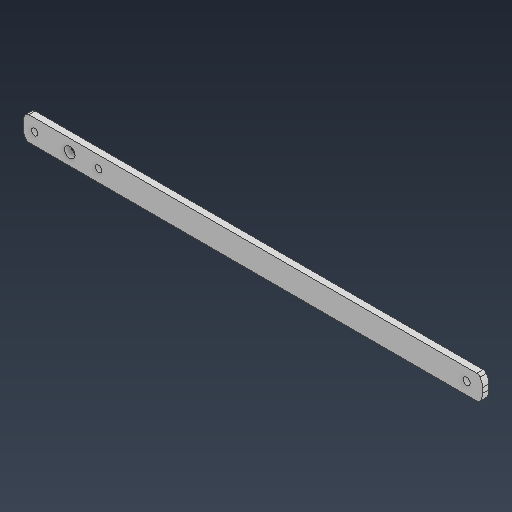
# Autodesk Inventor part: ДЛЯ ПОДВЕСА
Saved by Autodesk Inventor 2025 (Build 290162000, 162)
## iProperties
Created: 2025-03-11
Part Number: ДЛЯ ПОДВЕСА
Material: Типовые
Document SubType Name: Modeling
Designer: GameHD
Density: 1 g/cm^3
Appearance: По умолчанию
Author: GameHD
Autodesk Inventor part; units mm, degrees
ref_plane "YZ Plane" through (0, 0, 0) normal (1, 0, 0) x (0, 1, 0)
ref_plane "XZ Plane" through (0, 0, 0) normal (0, 1, 0) x (-1, 0, 0)
ref_plane "XY Plane" through (0, 0, 0) normal (0, 0, 1) x (1, 0, 0)
sketch "Эскиз1" plane through (0, 0, 0) normal (0, 0, 1) x (1, 0, 0)
  arc A0 (130.1731, 0.7623) -> (123.4106, 7.5248) centre (123.4106, 0.7623) ccw
  line L0 (-123.2839, 7.5248) -> (123.4106, 7.5248)
  arc A1 (-123.2839, 7.5248) -> (-130.0464, 0.7623) centre (-123.2839, 0.7623) ccw
  line L1 (-130.0464, -1.7127) -> (-130.0464, 0.7623)
  arc A2 (-130.0464, -1.7127) -> (-123.2839, -8.4752) centre (-123.2839, -1.7127) ccw
  line L2 (123.4106, -8.4752) -> (-123.2839, -8.4752)
  arc A3 (123.4106, -8.4752) -> (130.1731, -1.7127) centre (123.4106, -1.7127) ccw
  line L3 (130.1731, 0.7623) -> (130.1731, -1.7127)
  circle A4 centre (122.1731, -0.4752) radius 1.85
  circle A5 centre (-124.1763, -0.4762) radius 1.65
  circle A6 centre (-106.5766, -0.4757) radius 2.65
  circle A7 centre (-92.1769, -0.4756) radius 1.65
  line L4 (-73.2645, 4.044) -> (-78.5234, -4.9714)
  arc A8 (-71.5369, 4.044) -> (-73.2645, 4.044) centre (-72.4007, 3.5401) ccw
  line L5 (-66.2779, -4.9714) -> (-71.5369, 4.044)
  arc A9 (-67.1417, -6.4752) -> (-66.2779, -4.9714) centre (-67.1417, -5.4752) ccw
  line L6 (-77.6596, -6.4752) -> (-67.1417, -6.4752)
  arc A10 (-78.5234, -4.9714) -> (-77.6596, -6.4752) centre (-77.6596, -5.4752) ccw
  line L7 (-57.8267, 5.5248) -> (-68.3446, 5.5248)
  arc A11 (-56.9629, 4.0209) -> (-57.8267, 5.5248) centre (-57.8267, 4.5248) ccw
  line L8 (-62.2219, -4.9945) -> (-56.9629, 4.0209)
  arc A12 (-63.9495, -4.9945) -> (-62.2219, -4.9945) centre (-63.0857, -4.4906) ccw
  line L9 (-69.2084, 4.0209) -> (-63.9495, -4.9945)
  arc A13 (-68.3446, 5.5248) -> (-69.2084, 4.0209) centre (-68.3446, 4.5248) ccw
  line L10 (-54.634, 4.044) -> (-59.893, -4.9714)
  arc A14 (-52.9065, 4.044) -> (-54.634, 4.044) centre (-53.7703, 3.5401) ccw
  line L11 (-47.6475, -4.9714) -> (-52.9065, 4.044)
  arc A15 (-48.5113, -6.4752) -> (-47.6475, -4.9714) centre (-48.5113, -5.4752) ccw
  line L12 (-59.0292, -6.4752) -> (-48.5113, -6.4752)
  arc A16 (-59.893, -4.9714) -> (-59.0292, -6.4752) centre (-59.0292, -5.4752) ccw
  line L13 (-39.1963, 5.5248) -> (-49.7142, 5.5248)
  arc A17 (-38.3325, 4.0209) -> (-39.1963, 5.5248) centre (-39.1963, 4.5248) ccw
  line L14 (-43.5915, -4.9945) -> (-38.3325, 4.0209)
  arc A18 (-45.319, -4.9945) -> (-43.5915, -4.9945) centre (-44.4553, -4.4906) ccw
  line L15 (-50.578, 4.0209) -> (-45.319, -4.9945)
  arc A19 (-49.7142, 5.5248) -> (-50.578, 4.0209) centre (-49.7142, 4.5248) ccw
  line L16 (-36.0036, 4.044) -> (-41.2626, -4.9714)
  arc A20 (-34.2761, 4.044) -> (-36.0036, 4.044) centre (-35.1399, 3.5401) ccw
  line L17 (-29.0171, -4.9714) -> (-34.2761, 4.044)
  arc A21 (-29.8809, -6.4752) -> (-29.0171, -4.9714) centre (-29.8809, -5.4752) ccw
  line L18 (-40.3988, -6.4752) -> (-29.8809, -6.4752)
  arc A22 (-41.2626, -4.9714) -> (-40.3988, -6.4752) centre (-40.3988, -5.4752) ccw
  line L19 (-20.5659, 5.5248) -> (-31.0838, 5.5248)
  arc A23 (-19.7021, 4.0209) -> (-20.5659, 5.5248) centre (-20.5659, 4.5248) ccw
  line L20 (-24.9611, -4.9945) -> (-19.7021, 4.0209)
  arc A24 (-26.6886, -4.9945) -> (-24.9611, -4.9945) centre (-25.8249, -4.4906) ccw
  line L21 (-31.9476, 4.0209) -> (-26.6886, -4.9945)
  arc A25 (-31.0838, 5.5248) -> (-31.9476, 4.0209) centre (-31.0838, 4.5248) ccw
  line L22 (-17.3732, 4.044) -> (-22.6322, -4.9714)
  arc A26 (-15.6457, 4.044) -> (-17.3732, 4.044) centre (-16.5095, 3.5401) ccw
  line L23 (-10.3867, -4.9714) -> (-15.6457, 4.044)
  arc A27 (-11.2505, -6.4752) -> (-10.3867, -4.9714) centre (-11.2505, -5.4752) ccw
  line L24 (-21.7684, -6.4752) -> (-11.2505, -6.4752)
  arc A28 (-22.6322, -4.9714) -> (-21.7684, -6.4752) centre (-21.7684, -5.4752) ccw
  line L25 (-1.9355, 5.5248) -> (-12.4534, 5.5248)
  arc A29 (-1.0717, 4.0209) -> (-1.9355, 5.5248) centre (-1.9355, 4.5248) ccw
  line L26 (-6.3307, -4.9945) -> (-1.0717, 4.0209)
  arc A30 (-8.0582, -4.9945) -> (-6.3307, -4.9945) centre (-7.1945, -4.4906) ccw
  line L27 (-13.3172, 4.0209) -> (-8.0582, -4.9945)
  arc A31 (-12.4534, 5.5248) -> (-13.3172, 4.0209) centre (-12.4534, 4.5248) ccw
  line L28 (113.0396, 4.044) -> (107.7807, -4.9714)
  arc A32 (114.7672, 4.044) -> (113.0396, 4.044) centre (113.9034, 3.5401) ccw
  line L29 (120.0261, -4.9714) -> (114.7672, 4.044)
  arc A33 (119.1624, -6.4752) -> (120.0261, -4.9714) centre (119.1624, -5.4752) ccw
  line L30 (108.6444, -6.4752) -> (119.1624, -6.4752)
  arc A34 (107.7807, -4.9714) -> (108.6444, -6.4752) centre (108.6444, -5.4752) ccw
  line L31 (1.2572, 4.044) -> (-4.0018, -4.9714)
  arc A35 (2.9847, 4.044) -> (1.2572, 4.044) centre (2.121, 3.5401) ccw
  line L32 (8.2437, -4.9714) -> (2.9847, 4.044)
  arc A36 (7.3799, -6.4752) -> (8.2437, -4.9714) centre (7.3799, -5.4752) ccw
  line L33 (-3.138, -6.4752) -> (7.3799, -6.4752)
  arc A37 (-4.0018, -4.9714) -> (-3.138, -6.4752) centre (-3.138, -5.4752) ccw
  line L34 (16.6949, 5.5248) -> (6.177, 5.5248)
  arc A38 (17.5587, 4.0209) -> (16.6949, 5.5248) centre (16.6949, 4.5248) ccw
  line L35 (12.2997, -4.9945) -> (17.5587, 4.0209)
  arc A39 (10.5722, -4.9945) -> (12.2997, -4.9945) centre (11.436, -4.4906) ccw
  line L36 (5.3132, 4.0209) -> (10.5722, -4.9945)
  arc A40 (6.177, 5.5248) -> (5.3132, 4.0209) centre (6.177, 4.5248) ccw
  line L37 (98.4652, 4.0209) -> (103.7242, -4.9945)
  arc A41 (99.329, 5.5248) -> (98.4652, 4.0209) centre (99.329, 4.5248) ccw
  line L38 (109.847, 5.5248) -> (99.329, 5.5248)
  arc A42 (110.7107, 4.0209) -> (109.847, 5.5248) centre (109.847, 4.5248) ccw
  line L39 (105.4518, -4.9945) -> (110.7107, 4.0209)
  arc A43 (103.7242, -4.9945) -> (105.4518, -4.9945) centre (104.588, -4.4906) ccw
  line L40 (94.4092, 4.044) -> (89.1502, -4.9714)
  arc A44 (96.1368, 4.044) -> (94.4092, 4.044) centre (95.273, 3.5401) ccw
  line L41 (101.3957, -4.9714) -> (96.1368, 4.044)
  arc A45 (100.532, -6.4752) -> (101.3957, -4.9714) centre (100.532, -5.4752) ccw
  line L42 (90.014, -6.4752) -> (100.532, -6.4752)
  arc A46 (89.1502, -4.9714) -> (90.014, -6.4752) centre (90.014, -5.4752) ccw
  line L43 (19.8876, 4.044) -> (14.6286, -4.9714)
  arc A47 (21.6151, 4.044) -> (19.8876, 4.044) centre (20.7514, 3.5401) ccw
  line L44 (26.8741, -4.9714) -> (21.6151, 4.044)
  arc A48 (26.0103, -6.4752) -> (26.8741, -4.9714) centre (26.0103, -5.4752) ccw
  line L45 (15.4924, -6.4752) -> (26.0103, -6.4752)
  arc A49 (14.6286, -4.9714) -> (15.4924, -6.4752) centre (15.4924, -5.4752) ccw
  line L46 (35.3253, 5.5248) -> (24.8074, 5.5248)
  arc A50 (36.1891, 4.0209) -> (35.3253, 5.5248) centre (35.3253, 4.5248) ccw
  line L47 (30.9301, -4.9945) -> (36.1891, 4.0209)
  arc A51 (29.2026, -4.9945) -> (30.9301, -4.9945) centre (30.0664, -4.4906) ccw
  line L48 (23.9436, 4.0209) -> (29.2026, -4.9945)
  arc A52 (24.8074, 5.5248) -> (23.9436, 4.0209) centre (24.8074, 4.5248) ccw
  line L49 (79.8348, 4.0209) -> (85.0938, -4.9945)
  arc A53 (80.6986, 5.5248) -> (79.8348, 4.0209) centre (80.6986, 4.5248) ccw
  line L50 (91.2165, 5.5248) -> (80.6986, 5.5248)
  arc A54 (92.0803, 4.0209) -> (91.2165, 5.5248) centre (91.2165, 4.5248) ccw
  line L51 (86.8214, -4.9945) -> (92.0803, 4.0209)
  arc A55 (85.0938, -4.9945) -> (86.8214, -4.9945) centre (85.9576, -4.4906) ccw
  line L52 (75.7788, 4.044) -> (70.5198, -4.9714)
  arc A56 (77.5064, 4.044) -> (75.7788, 4.044) centre (76.6426, 3.5401) ccw
  line L53 (82.7653, -4.9714) -> (77.5064, 4.044)
  arc A57 (81.9015, -6.4752) -> (82.7653, -4.9714) centre (81.9015, -5.4752) ccw
  line L54 (71.3836, -6.4752) -> (81.9015, -6.4752)
  arc A58 (70.5198, -4.9714) -> (71.3836, -6.4752) centre (71.3836, -5.4752) ccw
  line L55 (38.518, 4.044) -> (33.259, -4.9714)
  arc A59 (40.2455, 4.044) -> (38.518, 4.044) centre (39.3818, 3.5401) ccw
  line L56 (45.5045, -4.9714) -> (40.2455, 4.044)
  arc A60 (44.6407, -6.4752) -> (45.5045, -4.9714) centre (44.6407, -5.4752) ccw
  line L57 (34.1228, -6.4752) -> (44.6407, -6.4752)
  arc A61 (33.259, -4.9714) -> (34.1228, -6.4752) centre (34.1228, -5.4752) ccw
  line L58 (53.9557, 5.5248) -> (43.4378, 5.5248)
  arc A62 (54.8195, 4.0209) -> (53.9557, 5.5248) centre (53.9557, 4.5248) ccw
  line L59 (49.5605, -4.9945) -> (54.8195, 4.0209)
  arc A63 (47.833, -4.9945) -> (49.5605, -4.9945) centre (48.6968, -4.4906) ccw
  line L60 (42.574, 4.0209) -> (47.833, -4.9945)
  arc A64 (43.4378, 5.5248) -> (42.574, 4.0209) centre (43.4378, 4.5248) ccw
  line L61 (61.2044, 4.0209) -> (66.4634, -4.9945)
  arc A65 (62.0682, 5.5248) -> (61.2044, 4.0209) centre (62.0682, 4.5248) ccw
  line L62 (72.5861, 5.5248) -> (62.0682, 5.5248)
  arc A66 (73.4499, 4.0209) -> (72.5861, 5.5248) centre (72.5861, 4.5248) ccw
  line L63 (68.191, -4.9945) -> (73.4499, 4.0209)
  arc A67 (66.4634, -4.9945) -> (68.191, -4.9945) centre (67.3272, -4.4906) ccw
  line L64 (57.1484, 4.044) -> (51.8894, -4.9714)
  arc A68 (58.876, 4.044) -> (57.1484, 4.044) centre (58.0122, 3.5401) ccw
  line L65 (64.1349, -4.9714) -> (58.876, 4.044)
  arc A69 (63.2711, -6.4752) -> (64.1349, -4.9714) centre (63.2711, -5.4752) ccw
  line L66 (52.7532, -6.4752) -> (63.2711, -6.4752)
  arc A70 (51.8894, -4.9714) -> (52.7532, -6.4752) centre (52.7532, -5.4752) ccw
  line L67 (122.1731, -0.4752) -> (92.1731, -0.4752)
  circle A71 centre (92.1731, -0.4752) radius 1.85
  arc A72 (100.1731, 0.7623) -> (93.4106, 7.5248) centre (93.4106, 0.7623) ccw
  arc A73 (93.4106, -8.4752) -> (100.1731, -1.7127) centre (93.4106, -1.7127) ccw
  line L68 (100.1731, 0.7623) -> (100.1731, -1.7127)
  point P0 (0, 0)
  point P1 (6.1731, -0.4752)
  point P2 (93.4106, -8.4752)
  dimension "d0" = 30
  constraints: 138 end point, 138 point on circle, 74 centre point, 1 coincident, 1 horizontal
  measures "d0" distance of L67.start L67.end
extrude "Выдавливание1" add sketch "Эскиз1" along normal blind 3.2 contours A72 A41 L37 L68 L67 L41 A44 L40 A71 A46 L42 A73 L2 A2 L1 A1 L0 | A72 L37 A41 | L42 A46 L40 A71 L67 L41 A73 | L41 L67 L68 A73 | L67 A71 L40 A44 L41 | A8 L5 A9 L6 A10 L4 | A11 L8 A12 L9 A13 L7 | A14 L11 A15 L12 A16 L10 | A17 L14 A18 L15 A19 L13 | A20 L17 A21 L18 A22 L16 | A23 L20 A24 L21 A25 L19 | A26 L23 A27 L24 A28 L22 | A29 L26 A30 L27 A31 L25 | A35 L32 A36 L33 A37 L31 | A38 L35 A39 L36 A40 L34 | A47 L44 A48 L45 A49 L43 | A50 L47 A51 L48 A52 L46 | A53 L50 A54 L51 A55 L49 | A56 L53 A57 L54 A58 L52 | A59 L56 A60 L57 A61 L55 | A62 L59 A63 L60 A64 L58 | A65 L62 A66 L63 A67 L61 | A68 L65 A69 L66 A70 L64
sketch "Эскиз2" plane through (0, 0, 3.2) normal (0, 0, 1) x (1, 0, 0)
  line L0 (100.1731, -1.7127) -> (100.1731, 0.7623) projected
  arc A0 (100.1731, 0.7623) -> (93.4106, 7.5248) centre (93.4106, 0.7623) ccw projected
  line L1 (93.4106, 7.5248) -> (-123.2839, 7.5248) projected
  arc A1 (-123.2839, 7.5248) -> (-130.0464, 0.7623) centre (-123.2839, 0.7623) ccw projected
  line L2 (-130.0464, 0.7623) -> (-130.0464, -1.7127) projected
  arc A2 (-130.0464, -1.7127) -> (-123.2839, -8.4752) centre (-123.2839, -1.7127) ccw projected
  line L3 (-123.2839, -8.4752) -> (93.4106, -8.4752) projected
  arc A3 (93.4106, -8.4752) -> (100.1731, -1.7127) centre (93.4106, -1.7127) ccw projected
  circle A4 centre (92.1731, -0.4752) radius 1.85 projected
  circle A5 centre (-106.5766, -0.4757) radius 2.65 projected
  circle A6 centre (-92.1769, -0.4756) radius 1.65 projected
  circle A7 centre (-124.1763, -0.4762) radius 1.65 projected
  line L4 (-128.0657, -6.4946) -> (127, -6.4946)
  line L5 (-124.1763, -0.4762) -> (-92.1769, -0.4756)
  line L6 (-130.0464, 5.5419) -> (126.9998, 5.5522)
  point P0 (0, 0)
  point P1 (-128.0659, 5.542)
  point P2 (98.1924, -6.4946)
  point P3 (-128.0678, 5.542)
  point P4 (98.1854, 5.551)
  constraints: 6 end point, 2 point on line, 2 symmetric about line, 1 horizontal, 1 point on circle
extrude "Выдавливание2" cut sketch "Эскиз2" against normal blind 3.2 contours A3 L3 A2 L4 | L6 A1 L1 A0
fillet "Сопряжение1" radius 2 4 edges at (-128.0657, -6.4946, 1.6) (-128.0678, 5.542, 1.6) (98.1854, 5.551, 1.6) (98.1924, -6.4946, 1.6)
